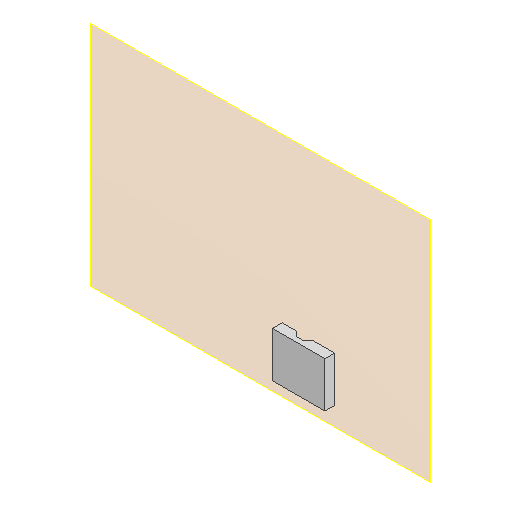
# Autodesk Inventor part: 20_Scanner_Fixation
Saved by Autodesk Inventor 2022 (Build 260153000, 153)
## iProperties
Created: 2022-09-19
Part Number: 20_Scanner_Fixation
Material: Generisch
Document SubType Name: Modeling
Designer: UC2
Density: 1 g/cm^3
Appearance: Vorgabe
Author: UC2
Autodesk Inventor part; units mm, degrees
ref_plane "YZ Plane" through (0, 0, 0) normal (1, 0, 0) x (0, 1, 0)
ref_plane "XZ Plane" through (0, 0, 0) normal (0, 1, 0) x (-1, 0, 0)
ref_plane "XY Plane" through (0, 0, 0) normal (0, 0, 1) x (1, 0, 0)
ref_plane "Arbeitsebene1" through (0, 0, 0) normal (0, 0, 1) x (1, 0, 0)
sketch "Skizze1" plane through (0, 0, 0) normal (0, 0, 1) x (1, 0, 0)
  line L0 (8.8222, -7.25) -> (-9.1, -7.25) projected
  line L1 (-9.1, -7.25) -> (-9.1, 29.75) projected
  line L2 (-9.1, 29.75) -> (45.9, 29.75) projected
  line L3 (45.9, 29.75) -> (45.9, -7.25) projected
  line L4 (45.9, -7.25) -> (27.9778, -7.25) projected
  line L5 (-63.9, -32.5058) -> (-63.9, -38.75) projected
  line L6 (63.9, -38.75) -> (63.9, 3.9837) projected
  line L7 (63.9, 3.9837) -> (56.9, 3.9837) projected
  line L8 (56.9, 3.9837) -> (56.9, 8.0046) projected
  spline S0 degree 2 poles (56.9, 8.0046) (47.4544, 9.25) (56.9, 10.4954) knots 0.408689 0.408689 0.408689 2.009633 2.009633 2.009633 weights 1.06106 1.156332 1.06106 projected
  line L9 (56.9, 10.4954) -> (56.9, 14.5163) projected
  line L10 (56.9, 14.5163) -> (63.9, 14.5163) projected
  arc A0 (63.9, 38.75) -> (59.9, 42.75) centre (59.9, 38.75) ccw projected
  line L11 (59.9, 42.75) -> (-59.9, 42.75) projected
  arc A1 (-59.9, 42.75) -> (-63.9, 38.75) centre (-59.9, 38.75) ccw projected
  line L12 (-63.9, 25.4963) -> (-55.9, 25.4963) projected
  line L13 (-55.9, 25.4963) -> (-55.9, 19.75) projected
  line L14 (-55.9, 19.75) -> (-18.9, 19.75) projected
  line L15 (-18.9, 19.75) -> (-18.9, 10.3274) projected
  spline S1 degree 2 poles (-18.9, 10.3274) (-11.6855, 9.25) (-18.9, 8.1726) knots 0.06387 0.06387 0.06387 0.952272 0.952272 0.952272 weights 1.010578 1.079212 1.010578 projected
  line L16 (-18.9, 8.1726) -> (-18.9, -1.25) projected
  line L17 (-18.9, -1.25) -> (-55.9, -1.25) projected
  line L18 (-55.9, -1.25) -> (-55.9, -6.9963) projected
  line L19 (-55.9, -6.9963) -> (-63.9, -6.9963) projected
  line L20 (-63.9, -6.9963) -> (-63.9, -22.9942) projected
  line L21 (14.75, -32.05) -> (21.15, -32.05)
  line L22 (21.15, -32.05) -> (21.15, -24.25)
  line L23 (21.15, -24.25) -> (14.75, -24.25)
  line L24 (14.75, -24.25) -> (14.75, -32.05)
  line L25 (8.8222, -20.5) -> (30.4914, -20.5)
  line L26 (30.4914, -20.5) -> (30.4914, -39.25)
  line L27 (30.4914, -39.25) -> (8.8222, -39.25)
  line L28 (8.8222, -39.25) -> (8.8222, -20.5)
  line L29 (63.9, 14.5163) -> (63.9, 38.75) projected
  circle A2 centre (5.4922, -12.0867) radius 1.4 projected
  circle A3 centre (17.95, -36.25) radius 1.4 projected
  circle A4 centre (-27.8589, -14.9953) radius 1.4 projected
  circle A5 centre (-42.2276, -36.25) radius 1.4 projected
  circle A6 centre (-42.2276, -19.25) radius 1.4 projected
  circle A7 centre (-27.8589, -39.949) radius 1.4 projected
  circle A8 centre (27.4914, -28.65) radius 1.4 projected
  circle A9 centre (32.285, -12.0867) radius 1.4 projected
  line L30 (-8.36, -23.75) -> (8.8222, -23.75) projected
  line L31 (8.8222, -23.75) -> (8.8222, -7.25) projected
  line L32 (27.9778, -7.25) -> (27.9778, -25.25) projected
  line L33 (27.9778, -25.25) -> (21.15, -25.25) projected
  line L34 (21.15, -25.25) -> (21.15, -32.05) projected
  line L35 (21.15, -32.05) -> (14.75, -32.05) projected
  line L36 (14.75, -32.05) -> (14.75, -31.75) projected
  line L37 (14.75, -31.75) -> (-8.36, -31.75) projected
  line L38 (-8.36, -31.75) -> (-8.36, -36.25) projected
  line L39 (-8.36, -36.25) -> (-23.36, -36.25) projected
  line L40 (-23.36, -33.75) -> (-23.36, -36.25) projected
  line L41 (-38.36, -33.75) -> (-23.36, -33.75) projected
  line L42 (-38.36, -33.75) -> (-38.36, -31.25) projected
  line L43 (-38.36, -31.25) -> (-41.36, -31.25) projected
  line L44 (-41.36, -31.25) -> (-41.36, -32.5058) projected
  line L45 (-41.36, -32.5058) -> (-63.9, -32.5058) projected
  arc A10 (-63.9, -38.75) -> (-59.9, -42.75) centre (-59.9, -38.75) ccw projected
  line L46 (-59.9, -42.75) -> (59.9, -42.75) projected
  arc A11 (59.9, -42.75) -> (63.9, -38.75) centre (59.9, -38.75) ccw projected
  line L47 (-63.9, 38.75) -> (-63.9, 25.4963) projected
  line L48 (-63.9, -22.9942) -> (-41.36, -22.9942) projected
  line L49 (-41.36, -22.9942) -> (-41.36, -24.25) projected
  line L50 (-41.36, -24.25) -> (-38.36, -24.25) projected
  line L51 (-38.36, -24.25) -> (-38.36, -21.75) projected
  line L52 (-38.36, -21.75) -> (-23.36, -21.75) projected
  line L53 (-23.36, -19.25) -> (-23.36, -21.75) projected
  line L54 (-23.36, -19.25) -> (-8.36, -19.25) projected
  line L55 (-8.36, -19.25) -> (-8.36, -23.75) projected
  point P0 (0, 0)
  point P1 (15.25, -24.75)
  dimension "d0" = 0.5
  constraints: 16 end point, 4 parallel, 2 horizontal, 2 perpendicular, 1 other
  measures "d0" distance from line of L23 point (15.25, -24.75)
extrude "Extrusion1" add sketch "Skizze1" along normal blind 4 contours L25 L32 L33 L22 L23 L24 L37 L28 | L25 L26 L27 L28 L37 L24 L21 L22 L33 L32 | L22 L21 L24 L23 | A3 | A8
sketch "Skizze2" plane through (0, 0, 0) normal (0, 0, -1) x (-1, 0, 0)
  line L0 (-8.8222, -39.25) -> (-30.4914, -39.25) projected
  line L1 (-8.8222, -20.5) -> (-8.8222, -39.25) projected
  line L2 (-30.4914, -20.5) -> (-8.8222, -20.5) projected
  line L3 (-30.4914, -39.25) -> (-30.4914, -20.5) projected
  line L4 (-14.75, -32.05) -> (-14.75, -24.25) projected
  line L5 (-8.8222, -20.5) -> (-8.8222, -39.25) projected
  line L6 (-14.75, -27.25) -> (-8.8222, -27.25)
  line L7 (-8.8222, -27.25) -> (-8.8222, -30.05)
  line L8 (-8.8222, -30.05) -> (-14.75, -30.05)
  line L9 (-14.75, -30.05) -> (-14.75, -27.25)
  line L10 (-14.75, -24.25) -> (-21.15, -24.25) projected
  line L11 (-30.4914, -20.5) -> (-8.8222, -20.5) projected
  line L12 (-19.35, -24.25) -> (-16.55, -24.25)
  line L13 (-16.55, -24.25) -> (-16.55, -20.5)
  line L14 (-16.55, -20.5) -> (-19.35, -20.5)
  line L15 (-19.35, -20.5) -> (-19.35, -24.25)
  point P0 (0, 0)
  constraints: 16 end point, 4 parallel, 4 point on line, 2 horizontal, 2 perpendicular
extrude "Extrusion2" cut sketch "Skizze2" against normal blind 2 contours L8 L4 L6 L1 | L2 L13 L10 L15
chamfer "Fase1" distance 1.8 angle 45 4 edges at (11.7861, -30.05, 0) (11.7861, -27.25, 0) (16.55, -22.375, 0) (19.35, -22.375, 0)
